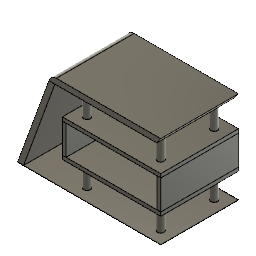
TV Stand (Autodesk Fusion 360 design; units mm, degrees)
description: TV  Stand
part number: TV-S-01
description: Box Top
part number: TV-S-01.001
description: Top
part number: TV-S-01.002
description: Box Right
part number: TV-S-01.003
description: Box Bottom
part number: TV-S-01.004
description: Bottom Plate
part number: TV-S-01.005
description: Box Left
part number: TV-S-01.006
description: Side
part number: TV-S-01.007
description: Tube
part number: TV-S-01.008
Autodesk Fusion 360 part; units mm, degrees
sketch "Volume" plane through (0, 0, 0) normal (0, 0, 1) x (1, 0, 0)
  line L0 (0, 0) -> (700, 0)
  line L1 (700, 0) -> (700, 450)
  line L2 (700, 450) -> (163.7866, 450)
  line L3 (163.7866, 450) -> (0, 0)
  dimension "d4" = 700
  dimension "d5" = 450
  dimension "d6" = 70
  measures "d4" distance of L0.start
  measures "d5" distance of L0 L2
  measures "d6" angle of L0 L3
extrude "Extrude1" add sketch "Volume" against normal blind 380 makes body 1
sketch "Shelf" plane through (0, 0, 0) normal (0, 0, 1) x (1, 0, 0)
  line L0 (163.7866, 450) -> (0, 0)
  line L1 (0, 0) -> (700, 0)
  line L2 (700, 0) -> (700, 450)
  line L3 (700, 450) -> (163.7866, 450)
  line L4 (700, 302) -> (220, 302)
  line L5 (220, 302) -> (220, 122)
  line L6 (220, 122) -> (700, 122)
  line L7 (700, 122) -> (700, 302)
  line L8 (238, 140) -> (682, 140)
  line L9 (682, 140) -> (682, 284)
  line L10 (682, 284) -> (238, 284)
  line L11 (238, 284) -> (238, 140)
  line L12 (238, 284) -> (220, 284)
  line L13 (238, 140) -> (220, 140)
  line L14 (682, 284) -> (700, 284)
  line L15 (682, 140) -> (700, 140)
  line L16 (700, 422) -> (560, 422) construction
  line L17 (700, 2) -> (585.0967, 2) construction
  dimension "d12" = 18
  dimension "d53" = 28
  dimension "d54" = 2
  dimension "d56" = 120
  dimension "d57" = 120
  dimension "d58" = 220
  measures "d12" distance of L6
  measures "d53" distance of L3 L16
  measures "d54" distance of L1 L17
  measures "d56" distance of L4 L16
  measures "d57" distance of L6 L17
extrude "Extrude2" add sketch "Shelf" against normal up to surface (380 mm away) separate body contours L2 L4 L5 L7 L10 L12 L14 makes body 2
extrude "Extrude3" add sketch "Shelf" against normal up to surface (380 mm away) separate body contours L2 L7 L9 L14 L15 makes body 3
extrude "Extrude4" add sketch "Shelf" against normal up to surface (380 mm away) separate body contours L2 L5 L6 L7 L8 L13 L15 makes body 4
extrude "Extrude5" add sketch "Shelf" against normal up to surface (380 mm away) separate body contours L5 L11 L12 L13 makes body 5
sketch "Bottom Plate" plane through (0, 0, 0) normal (0, 0, 1) x (1, 0, 0)
  line L0 (700, 0) -> (0, 0)
  line L1 (163.7866, 450) -> (0, 0)
  line L2 (700, 450) -> (163.7866, 450) construction
  line L3 (700, 0) -> (0, 0)
  line L4 (0, 0) -> (0, 2)
  line L5 (0, 2) -> (700, 2)
  line L6 (700, 2) -> (700, 0)
  dimension "d23" = 2
extrude "Extrude6" add sketch "Bottom Plate" against normal up to surface (380 mm away) separate body contours L0 L1 L3 L5 L6 makes body 6
sketch "Top" plane through (0, 0, 0) normal (0, 0, 1) x (1, 0, 0)
  line L0 (163.7866, 450) -> (0, 0)
  line L1 (163.7866, 450) -> (153.5954, 422)
  line L2 (700, 0) -> (700, 450)
  line L3 (700, 422) -> (153.5954, 422)
  line L4 (700, 450) -> (163.7866, 450)
  line L5 (700, 450) -> (700, 422)
  dimension "d35" = 28
  measures "d35" distance of L3 L4
extrude "Extrude9" add sketch "Top" against normal up to surface (380 mm away) separate body makes body 7
sketch "Side" plane through (0, 0, 0) normal (0, 0, 1) x (1, 0, 0)
  line L0 (700, 422) -> (153.5954, 422)
  line L1 (0.7279, 2) -> (700, 2)
  line L2 (183.3924, 422) -> (30.5249, 2)
  line L3 (163.7866, 450) -> (0, 0)
  dimension "d38" = 28
  measures "d38" distance of L2 L3
extrude "Extrude10" add sketch "Side" against normal up to surface (380 mm away) separate body makes body 8
fillet "Fillet2" radius 38 1 edges at (163.7866, 450, -190) on bodies 7
chamfer "Chamfer1" distance 20 distance2 28 1 edges at (700, 422, -190) measured on face at (517.8651, 422, -126.6667) on bodies 7
sketch "Sketch8" plane through (0, 302, 0) normal (0, 1, 0) x (-1, 0, 0)
  line L0 (-700, -380) -> (-220, -380)
  line L1 (-220, -380) -> (-220, 0)
  line L2 (-220, 0) -> (-700, 0)
  line L3 (-700, 0) -> (-700, -380)
  line L4 (-280, -320) -> (-640, -320) construction
  line L5 (-640, -320) -> (-640, -60) construction
  line L6 (-640, -60) -> (-280, -60) construction
  line L7 (-280, -60) -> (-280, -320) construction
  circle A0 centre (-640, -60) radius 16
  circle A1 centre (-640, -60) radius 15
  dimension "d44" = 60
  dimension "d45" = 60
  dimension "d47" = 60
  dimension "d48" = 60
  dimension "d49" = 32
  dimension "d50" = 1
  measures "d44" distance of L3 L5
  measures "d45" distance of L1 L7
  measures "d47" distance of L0 L4
  measures "d48" distance of L2 L6
  measures "d49" diameter of A0
extrude "Extrude11" add sketch "Sketch8" along normal up to surface (120 mm away) separate body contours A0 makes body 9
copy_body "Body->Comp1" bodies 2 removing the originals makes body 10 in component "Box Top"
copy_body "Body->Comp2" bodies 7 removing the originals makes body 11 in component "Top"
copy_body "Body->Comp3" bodies 3 removing the originals makes body 12 in component "Box Right"
copy_body "Body->Comp4" bodies 4 removing the originals makes body 13 in component "Box Bottom"
copy_body "Body->Comp5" bodies 6 removing the originals makes body 14 in component "Bottom Plate"
copy_body "Body->Comp6" bodies 5 removing the originals makes body 15 in component "Box Left"
copy_body "Body->Comp7" bodies 8 removing the originals makes body 16 in component "Side"
copy_body "Body->Comp8" bodies 9 removing the originals makes body 17 in component "Tube"
pattern_linear "R-Pattern1" [suppressed]
pattern_linear "R-Pattern2" [suppressed]
component "Box Top" placed x (1, 0, 0) y (0, 1, 0) z (0, 0, 1) at (0, 0, 0)
component "Top" placed x (1, 0, 0) y (0, 1, 0) z (0, 0, 1) at (0, 0, 0)
component "Box Right" placed x (1, 0, 0) y (0, 1, 0) z (0, 0, 1) at (0, 0, 0)
component "Box Bottom" placed x (1, 0, 0) y (0, 1, 0) z (0, 0, 1) at (0, 0, 0)
component "Bottom Plate" placed x (1, 0, 0) y (0, 1, 0) z (0, 0, 1) at (0, 0, 0)
component "Box Left" placed x (1, 0, 0) y (0, 1, 0) z (0, 0, 1) at (0, 0, 0)
component "Side" placed x (1, 0, 0) y (0, 1, 0) z (0, 0, 1) at (0, 0, 0)
component "Tube" placed x (1, 0, 0) y (0, 1, 0) z (0, 0, 1) at (0, 0, 0)
component "Tube" placed x (1, 0, 0) y (0, 1, 0) z (0, 0, 1) at (0, 0, -260)
component "Tube" placed x (1, 0, 0) y (0, 1, 0) z (0, 0, 1) at (-360, 0, 0)
component "Tube" placed x (1, 0, 0) y (0, 1, 0) z (0, 0, 1) at (-360, 0, -260)
component "Tube" placed x (1, 0, 0) y (0, 1, 0) z (0, 0, 1) at (0, -300, 0)
component "Tube" placed x (1, 0, 0) y (0, 1, 0) z (0, 0, 1) at (0, -300, -260)
component "Tube" placed x (1, 0, 0) y (0, 1, 0) z (0, 0, 1) at (-360, -300, 0)
component "Tube" placed x (1, 0, 0) y (0, 1, 0) z (0, 0, 1) at (-360, -300, -260)
hidden bodies 1
equation "Height = 450 mm"
equation "Width = 700 mm"
equation "Depth = 380 mm"
equation "d4 = Width"
equation "d5 = Height"
equation "d7 = -Depth"
equation "d45 = d44"
equation "d57 = d56"
named bodies: "Volume", "Box Top", "Box Right", "Box Bottom", "Box Left", "Bottom Plate", "Top", "Side", "Tube"
